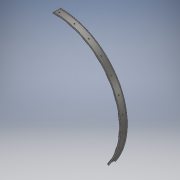
# Autodesk Inventor part: support2
Saved by Autodesk Inventor 2019 (Build 230136000, 136)
## iProperties
Created: 2019-02-24
Part Number: support2
Material: Stainless Steel
Document SubType Name: Modeling
Designer: gaincarlo
Density: 8 g/cm^3
Appearance: Semi-Polished
Author: gaincarlo
Autodesk Inventor part; units mm, degrees
ref_plane "YZ Plane" through (0, 0, 0) normal (1, 0, 0) x (0, 1, 0)
ref_plane "XZ Plane" through (0, 0, 0) normal (0, 1, 0) x (-1, 0, 0)
ref_plane "XY Plane" through (0, 0, 0) normal (0, 0, 1) x (1, 0, 0)
sketch "Sketch1" plane through (0, 0, 0) normal (0, 0, 1) x (1, 0, 0)
  arc A0 (491.4912, -344.1459) -> (0, 600) centre (0, 0) ccw
  line L0 (0, 0) -> (0, 600) construction
  line L1 (0, 0) -> (491.4912, -344.1459) construction
  arc A1 (481.6614, -337.2629) -> (0, 588) centre (0, 0) ccw
  line L2 (0, 600) -> (0, 588)
  line L3 (481.6614, -337.2629) -> (491.4912, -344.1459)
  dimension "d0" = 1200
  dimension "d1" = 125
  dimension "d2" = 1176
  constraints: 8 end point, 4 point on circle, 3 point on line, 2 centre point, 1 coincident, 1 collinear, 1 vertical
  measures "d0" diameter of A0
  measures "d1" angle of L1 L0
  measures "d2" diameter of A1
extrude "Extrusion1" add sketch "Sketch1" along normal blind 60
sketch "Sketch2" plane through (0, 588, 0) normal (-1, 0, 0) x (0, 0, 1)
  line L0 (0, 12) -> (60, 12) projected
  line L1 (60, 12) -> (60, 0) projected
  line L2 (60, 0) -> (0, 0) projected
  line L3 (0, 0) -> (0, 12) projected
  line L4 (1, 12) -> (1, 3)
  line L5 (1, 3) -> (59, 3)
  line L6 (59, 3) -> (59, 12)
  line L7 (-12, -588) -> (72, -588) projected
  point P0 (0, -588)
  constraints: 6 end point, 2 point on line
revolve "Revolution1" cut sketch "Sketch2" angle 360 about axis through (0, 0, -10) along (0, 0, 1) contours L0 L6 L5 L4
sketch "Sketch3" plane through (0, 0, 60) normal (0, 0, 1) x (1, 0, 0)
  arc A0 (481.6614, -337.2629) -> (0, 588) centre (0, 0) ccw projected
  line L0 (479.9667, -336.2009) -> (511.8289, -285.3599)
  line L1 (511.8289, -285.3599) -> (513.5236, -286.422)
  line L2 (513.5236, -286.422) -> (481.6614, -337.2629)
  line L3 (479.9667, -336.2009) -> (481.6614, -337.2629)
  dimension "d7" = 2
  dimension "d8" = 60
  constraints: 8 end point, 2 perpendicular, 1 parallel, 1 point on circle
  measures "d7" distance of L0.end L1.end
  measures "d8" distance of L0.start L0.end
extrude "Extrusion2" add sketch "Sketch3" against normal blind 60 contours L3 L0 L1 L2
sketch "Sketch4" plane through (511.8289, -285.3599, 0) normal (-0.8473493, 0.5310359, 0) x (0, 0, 1)
  circle A0 centre (30, -30) radius 5
  line L0 (60, 0) -> (60, -60) construction
  line L1 (60, 0) -> (0, 0) construction
  line L2 (0, -60) -> (0, 0) construction
  line L3 (60, -60) -> (0, -60) construction
  line L4 (0, -60) -> (60, 0) construction
  point P0 (0, -30)
  dimension "d14" = 10
  constraints: 2 end point, 1 centre point, 1 coincident, 1 midpoint
  measures "d14" diameter of A0
extrude "Extrusion3" cut sketch "Sketch4" against normal through all
pattern_circular "Circular Pattern1" count 10 over 120 about axis through (0, 0, -10) along (0, 0, 1) of "Extrusion2", "Extrusion3"
body "Solid1"
